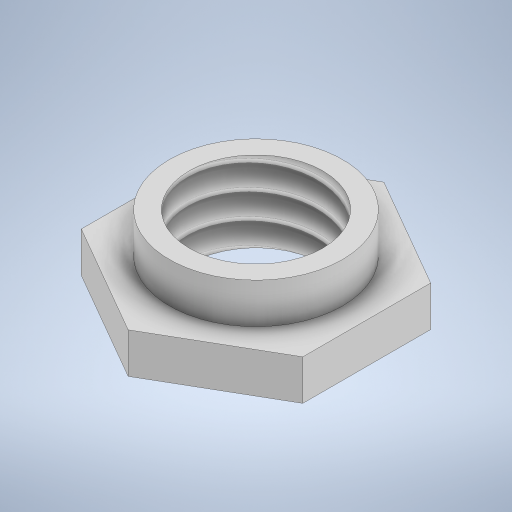
# Autodesk Inventor part: Pot Adaptor
Saved by Autodesk Inventor 2023 (Build 270158030, 158C)
## iProperties
Created: 2022-12-30
Part Number: Pot Adaptor
Material: Generic
Document SubType Name: Modeling
Designer: Imogen Heard
Density: 1 g/cm^3
Appearance: Default
Author: Imogen Heard
Autodesk Inventor part; units mm, degrees
ref_plane "YZ Plane" through (0, 0, 0) normal (1, 0, 0) x (0, 1, 0)
ref_plane "XZ Plane" through (0, 0, 0) normal (0, 1, 0) x (-1, 0, 0)
ref_plane "XY Plane" through (0, 0, 0) normal (0, 0, 1) x (1, 0, 0)
sketch "Sketch1" plane through (0, 0, 0) normal (0, 1, 0) x (-1, 0, 0)
  line L0 (-5.5, 3.1754) -> (0, 6.3509)
  line L1 (0, 6.3509) -> (5.5, 3.1754)
  line L2 (5.5, 3.1754) -> (5.5, -3.1754)
  line L3 (5.5, -3.1754) -> (0, -6.3509)
  line L4 (0, -6.3509) -> (-5.5, -3.1754)
  line L5 (-5.5, -3.1754) -> (-5.5, 3.1754)
  point P0 (0, 0)
  point P1 (0, 0)
  dimension "d0" = 11
  constraints: 12 end point, 1 coincident, 1 vertical, 13 other
  measures "d0" distance between parallel lines of L5 L2
extrude "Extrusion1" add sketch "Sketch1" along normal blind 2
sketch "Sketch2" plane through (0, 2, 0) normal (0, 1, 0) x (1, 0, 0)
  circle A0 centre (0, 0) radius 4.3
  dimension "d3" = 8.6
  constraints: 1 centre point, 1 coincident
  measures "d3" diameter of A0
extrude "Extrusion2" add sketch "Sketch2" along normal blind 2
sketch "Sketch3" plane through (0, 4, 0) normal (0, 1, 0) x (1, 0, 0)
  circle A0 centre (0, 0) radius 4
  circle A1 centre (0, 0) radius 4.3 projected
  dimension "d6" = 8
  constraints: 1 centre point, 1 concentric
  measures "d6" diameter of A0
hole "Hole1" at (0, 4, 0) direction (0, -1, 0) diameter 6.647 end through all thread size "M8x1.25" class "6H" standard "ISO Metric profile"
body "Solid1"
